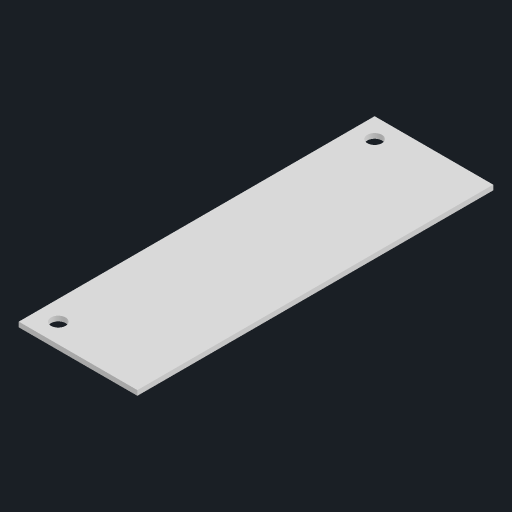
# Autodesk Inventor part: underside
Saved by Autodesk Inventor 2024.2 (Build 282272000, 272)
## iProperties
Created: 2023-12-14
Part Number: underside
Material: Generic
Document SubType Name: Sheet Metal
Designer: reima
Density: 1 g/cm^3
Sheet Metal Rule: Default
Appearance: Default
Author: reima
Autodesk Inventor part; units mm, degrees
ref_plane "YZ Plane" through (0, 0, 0) normal (1, 0, 0) x (0, 1, 0)
ref_plane "XZ Plane" through (0, 0, 0) normal (0, 1, 0) x (-1, 0, 0)
ref_plane "XY Plane" through (0, 0, 0) normal (0, 0, 1) x (1, 0, 0)
sketch "Sketch4" plane through (0, 0, 0) normal (0, 1, 0) x (-1, 0, 0)
  line L0 (-6.6563, 17.1443) -> (-44.7563, 17.1443)
  line L1 (-44.7563, 17.1443) -> (-44.7563, -97.1557)
  line L2 (-44.7563, -97.1557) -> (-6.6563, -97.1557)
  line L3 (-6.6563, -97.1557) -> (-6.6563, 17.1443)
  circle A0 centre (-13.0063, 10.7943) radius 2.3368
  circle A1 centre (-13.0063, -90.8057) radius 2.3368
  point P0 (0, 0)
  dimension "d41" = 38.1
  dimension "d42" = 114.3
  dimension "d43" = 4.6736
  dimension "d44" = 4.6736
  dimension "d45" = 6.35
  dimension "d46" = 6.35
  dimension "d47" = 6.35
  dimension "d48" = 6.35
  measures "d41" distance of L2.end L1.end
  measures "d42" distance of L1.end L0.end
  measures "d43" diameter of A0
  measures "d44" diameter of A1
  measures "d45" distance from line of L3 A0.centre
  measures "d46" distance from line of L0 A0.centre
  measures "d47" distance from line of L3 A1.centre
  measures "d48" distance from line of L2 A1.centre
extrude "Plate4" add sketch "Sketch4" along normal blind 1.5875
equation "\"d49\" = Thickness"
equation "\"BendRadius\" = Thickness"
equation "\"BendReliefWidth\" = Thickness"
equation "\"BendReliefDepth\" = 0.5 * Thickness"
equation "\"CornerReliefSize\" = 4 * Thickness"
equation "\"MinimumRemnant\" = 2 * Thickness"
equation "\"TransitionRadius\" = BendRadius"
equation "\"JacobiRadiusSize\" = BendRadius"
equation "\"GapSize\" = Thickness"
equation "\"Thickness\" = 1.5875"
body "Solid2"
